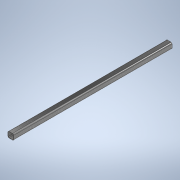
# Autodesk Inventor part: Horquilla_Perfil
Saved by Autodesk Inventor 2022.1 (Build 261234000, 234)
## iProperties
Created: 2021-09-10
Part Number: Horquilla_Perfil
Material: Genérico
Document SubType Name: Modeling
Designer: seb_0
Density: 1 g/cm^3
Appearance: Acero galvanizado
Author: seb_0
Autodesk Inventor part; units mm, degrees
ref_plane "YZ Plane" through (0, 0, 0) normal (1, 0, 0) x (0, 1, 0)
ref_plane "XZ Plane" through (0, 0, 0) normal (0, 1, 0) x (-1, 0, 0)
ref_plane "XY Plane" through (0, 0, 0) normal (0, 0, 1) x (1, 0, 0)
sketch "Boceto1" plane through (0, 0, 0) normal (0, 0, 1) x (1, 0, 0)
  line L0 (-10, 0) -> (-40, 0)
  line L1 (-50, 10) -> (-50, 40)
  line L2 (-40, 50) -> (-10, 50)
  line L3 (0, 40) -> (0, 10)
  arc A0 (-40, 50) -> (-50, 40) centre (-40, 40) ccw
  arc A1 (0, 40) -> (-10, 50) centre (-10, 40) ccw
  arc A2 (-50, 10) -> (-40, 0) centre (-40, 10) ccw
  arc A3 (-10, 0) -> (0, 10) centre (-10, 10) ccw
  line L4 (-10, 46) -> (-40, 46)
  arc A4 (-40, 46) -> (-46, 40) centre (-40, 40) ccw
  line L5 (-46, 40) -> (-46, 10)
  arc A5 (-46, 10) -> (-40, 4) centre (-40, 10) ccw
  line L6 (-40, 4) -> (-10, 4)
  arc A6 (-10, 4) -> (-4, 10) centre (-10, 10) ccw
  line L7 (-4, 10) -> (-4, 40)
  arc A7 (-4, 40) -> (-10, 46) centre (-10, 40) ccw
  point P0 (0, 0)
  point P1 (-50, 50)
  point P2 (-50, 0)
  point P3 (0, 50)
  dimension "d0" = 50
  dimension "d1" = 50
  dimension "d2" = 10
  dimension "d3" = 10
  dimension "d4" = 10
  dimension "d5" = 10
  dimension "d6" = 4
  constraints: 16 end point, 16 point on circle, 8 centre point, 8 point on line, 8 tangent, 4 parallel, 2 perpendicular, 1 horizontal, 7 other
  measures "d0" distance of point (-50, 0) point (-50, 50)
  measures "d1" distance of point (-50, 50) point (0, 50)
  measures "d2" radius of A0
  measures "d3" radius of A1
  measures "d4" radius of A2
  measures "d5" radius of A3
  measures "d6" distance between parallel lines of L2 L4
extrude "Extrusión1" add sketch "Boceto1" against normal blind 1350
